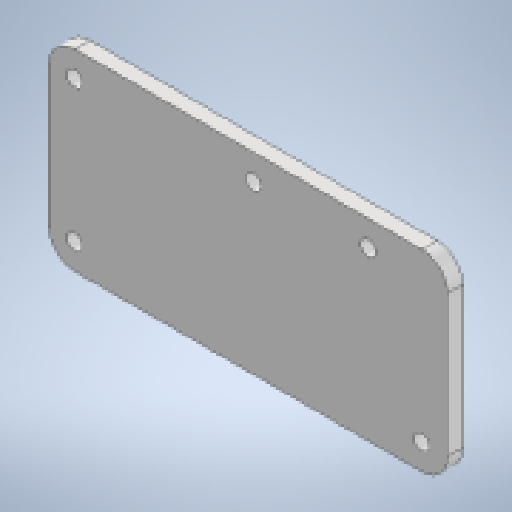
# Autodesk Inventor part: CaseCover
Saved by Autodesk Inventor 2025.2 (Build 292293000, 293)
## iProperties
Created: 2026-02-21
Part Number: CaseCover
Material: 一般
Document SubType Name: Modeling
Designer: naka6
Density: 1 g/cm^3
Appearance: 既定
Author: naka6
Autodesk Inventor part; units mm, degrees
ref_plane "YZ Plane" through (0, 0, 0) normal (1, 0, 0) x (0, 1, 0)
ref_plane "XZ Plane" through (0, 0, 0) normal (0, 1, 0) x (-1, 0, 0)
ref_plane "XY Plane" through (0, 0, 0) normal (0, 0, 1) x (1, 0, 0)
sketch "スケッチ1" plane through (0, 0, 0) normal (0, 0, 1) x (1, 0, 0)
  line L0 (9.4222, 72.3) -> (45.5, 72.3) projected
  arc A0 (50.5, 67.3) -> (45.5, 72.3) centre (45.5, 67.3) ccw projected
  line L1 (50.5, 67.3) -> (50.5, 43.9148) projected
  arc A1 (45.8359, 41.4187) -> (50.5, 43.9148) centre (47.5, 43.9148) ccw projected
  line L2 (45.8359, 41.4187) -> (7.7581, 66.8038) projected
  arc A2 (9.4222, 72.3) -> (7.7581, 66.8038) centre (9.4222, 69.3) ccw projected
  line L3 (31.5778, 32.3) -> (-4.5, 32.3) projected
  arc A3 (-9.5, 37.3) -> (-4.5, 32.3) centre (-4.5, 37.3) ccw projected
  line L4 (-9.5, 37.3) -> (-9.5, 60.6852) projected
  arc A4 (-4.8359, 63.1813) -> (-9.5, 60.6852) centre (-6.5, 60.6852) ccw projected
  line L5 (-4.8359, 63.1813) -> (33.2419, 37.7962) projected
  arc A5 (31.5778, 32.3) -> (33.2419, 37.7962) centre (31.5778, 35.3) ccw projected
  arc A6 (50.5, -32.7) -> (55.5, -27.7) centre (50.5, -27.7) ccw projected
  line L6 (55.5, -27.7) -> (55.5, 77.3) projected
  line L7 (55.5, 77.3) -> (-14.5, 77.3) projected
  line L8 (-14.5, 77.3) -> (-14.5, 27.3) projected
  line L9 (-14.5, 27.3) -> (-22.2876, 1.4419) projected
  arc A7 (-16.3774, 4.8724) -> (-22.2876, 1.4419) centre (-17.5, 0) ccw projected
  arc A8 (-16.3774, 4.8724) -> (-12.2872, 6.71) centre (-15.5442, 8.4886) ccw projected
  arc A9 (-7.5, 11.8216) -> (-12.2872, 6.71) centre (0, 0) ccw projected
  line L10 (-7.5, 11.8216) -> (-7.5, 18.5) projected
  arc A10 (-1.5, 24.5) -> (-7.5, 18.5) centre (-1.5, 18.5) ccw projected
  line L11 (-1.5, 24.5) -> (42.5, 24.5) projected
  arc A11 (48.5, 18.5) -> (42.5, 24.5) centre (42.5, 18.5) ccw projected
  line L12 (48.5, 18.5) -> (48.5, -8.5) projected
  line L13 (48.5, -8.5) -> (39.5, -8.5) projected
  arc A12 (31.5, -0.5) -> (39.5, -8.5) centre (39.5, -0.5) ccw projected
  line L14 (31.5, -0.5) -> (31.5, 8.5) projected
  line L15 (31.5, 8.5) -> (11.1243, 8.5) projected
  arc A13 (12.2844, 6.7152) -> (11.1243, 8.5) centre (0, 0) ccw projected
  arc A14 (12.2844, 6.7152) -> (16.3816, 4.8733) centre (15.5493, 8.5) ccw projected
  arc A15 (17.5, -5) -> (16.3816, 4.8733) centre (17.5, 0) ccw projected
  line L16 (17.5, -5) -> (10.0995, -5) projected
  arc A16 (8.3431, -3.9565) -> (10.0995, -5) centre (10.0995, -3) ccw projected
  arc A17 (8.3431, -3.9565) -> (-8.3431, -3.9565) centre (0, -8.5) ccw projected
  arc A18 (-10.0995, -5) -> (-8.3431, -3.9565) centre (-10.0995, -3) ccw projected
  line L17 (-10.0995, -5) -> (-17.5, -5) projected
  arc A19 (-22.5, 0) -> (-17.5, -5) centre (-17.5, 0) ccw projected
  line L18 (-22.5, 0) -> (-22.5, -27.7) projected
  arc A20 (-22.5, -27.7) -> (-17.5, -32.7) centre (-17.5, -27.7) ccw projected
  line L19 (-17.5, -32.7) -> (50.5, -32.7) projected
  circle A21 centre (-17.5, -27.7) radius 1.9 projected
  circle A22 centre (50.5, -27.7) radius 1.9 projected
  line L20 (55.5, -32.7) -> (-22.5, -32.7)
  line L21 (-22.5, -32.7) -> (-22.5, 5)
  line L22 (-22.5, 5) -> (55.5, 5)
  line L23 (55.5, 5) -> (55.5, -32.7)
  arc A23 (-16.3774, 4.8724) -> (-17.5, -5) centre (-17.5, 0) ccw projected
  point P0 (0, 0)
  point P1 (-17.5, 5)
  constraints: 8 end point, 2 parallel, 2 point on line, 1 horizontal, 1 perpendicular, 1 tangent
extrude "押し出し1" add sketch "スケッチ1" along normal blind 3 contours L19 A20 L18 A19 L17 A18 A17 A16 L16 A15 L22 L14 A12 L13 L12 L6 A6 | L12 L13 A12 L14 L22 | A23 A7 A8 L22 A14 A15 L16 A16 A17 A18 L17 A19 | A15 A14 L22 | L22 A8 A7 | A21 | A22
fillet "フィレット1" radius 5 1 edges at (55.5, 5, 1.5)
sketch "スケッチ2" plane through (0, 0, 3) normal (0, 0, 1) x (1, 0, 0)
  circle A0 centre (-17.5, 0) radius 1.4 projected
  circle A1 centre (-17.5, -27.7) radius 1.4 projected
  circle A2 centre (17.5, 0) radius 1.4 projected
  circle A3 centre (40, 0) radius 1.35 projected
  circle A4 centre (50.5, -27.7) radius 1.4 projected
  point P0 (0, 0)
hole "穴1" at (40, 0, 3) at (17.5, 0, 3) at (-17.5, 0, 3) at (-17.5, -27.7, 3) at (50.5, -27.7, 3) direction (0, 0, -1) diameter 3 end through all
